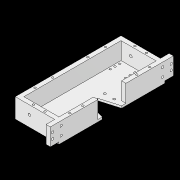
# Autodesk Inventor part: AfterComp1Chassis
Saved by Autodesk Inventor 2022 (Build 260153000, 153)
## iProperties
Created: 2021-02-15
Part Number: AfterComp1Chassis
Material: UHMW, White
Document SubType Name: Modeling
Designer: Esketitttttt
Density: 0.94 g/cm^3
Appearance: Smooth - White
Mass: 85.6235 g
Surface Area: 428.67 cm^2
Volume: 91.0888 cm^3
ThreadingScrew: 0.116 in
ThroughScrew: 0.138 in
Author: Esketitttttt
Autodesk Inventor part; units mm, degrees
ref_plane "YZ Plane" through (0, 0, 0) normal (1, 0, 0) x (0, 1, 0)
ref_plane "XZ Plane" through (0, 0, 0) normal (0, 1, 0) x (-1, 0, 0)
sketch "BasePlan" plane through (0, 0, 0) normal (0, 1, 0) x (-1, 0, 0)
  line L0 (0, 0) -> (-51.64, 0)
  line L1 (-51.64, 0) -> (-51.64, -28.5122)
  line L2 (-51.64, -28.5122) -> (0, -28.5122)
  line L3 (0, -28.5122) -> (0, 0)
  line L4 (0, 0) -> (-28.78, 0)
  line L5 (-28.78, 0) -> (-28.78, 57.15)
  line L6 (-28.78, 57.15) -> (0, 57.15)
  line L7 (0, 57.15) -> (0, 0)
  line L8 (-28.78, 57.15) -> (-51.64, 57.15)
  line L9 (-51.64, 57.15) -> (-51.64, 0)
  line L10 (-51.64, 0) -> (-28.78, 0)
  line L11 (-28.78, 0) -> (-28.78, 57.15)
  line L12 (0, 0) -> (0, -14.2561)
  line L13 (0, -14.2561) -> (8.9825, -14.2561) construction
  line L14 (-28.78, -28.5122) -> (-28.78, -85.6622)
  line L15 (-28.78, -85.6622) -> (0, -85.6622)
  line L16 (0, -85.6622) -> (0, -28.5122)
  line L17 (-28.78, -85.6622) -> (-51.64, -85.6622)
  line L18 (-51.64, -85.6622) -> (-51.64, -28.5122)
  line L19 (0, -85.6622) -> (6.35, -85.6622) construction
  line L20 (6.35, -85.6622) -> (6.35, -92.0122) construction
  line L21 (6.35, -92.0122) -> (0, -92.0122) construction
  line L22 (0, -92.0122) -> (0, -85.6622) construction
  line L23 (0, 57.15) -> (6.35, 57.15) construction
  line L24 (6.35, 57.15) -> (6.35, 63.5) construction
  line L25 (6.35, 63.5) -> (0, 63.5) construction
  line L26 (0, 63.5) -> (0, 57.15) construction
  line L27 (-51.64, -85.6622) -> (-57.99, -85.6622) construction
  line L28 (-57.99, -85.6622) -> (-57.99, -92.0122) construction
  line L29 (-57.99, -92.0122) -> (-51.64, -92.0122) construction
  line L30 (-51.64, -92.0122) -> (-51.64, -85.6622) construction
  line L31 (-51.64, 57.15) -> (-57.99, 57.15) construction
  line L32 (-57.99, 57.15) -> (-57.99, 63.5) construction
  line L33 (-57.99, 63.5) -> (-51.64, 63.5) construction
  line L34 (-51.64, 63.5) -> (-51.64, 57.15) construction
  line L35 (-57.99, 63.5) -> (-51.64, 63.5)
  line L36 (-51.64, 63.5) -> (-51.64, 0)
  line L37 (-51.64, 0) -> (-57.99, 0)
  line L38 (-57.99, 0) -> (-57.99, 63.5)
  line L39 (6.35, 63.5) -> (0, 63.5)
  line L40 (0, 63.5) -> (0, -92.0122)
  line L41 (0, -92.0122) -> (6.35, -92.0122)
  line L42 (6.35, -92.0122) -> (6.35, 63.5)
  line L43 (-51.64, 63.5) -> (0, 63.5)
  line L44 (0, 63.5) -> (0, 57.15)
  line L45 (0, 57.15) -> (-51.64, 57.15)
  line L46 (-51.64, 57.15) -> (-51.64, 63.5)
  line L47 (-51.64, -85.6622) -> (0, -85.6622)
  line L48 (0, -85.6622) -> (0, -92.0122)
  line L49 (0, -92.0122) -> (-51.64, -92.0122)
  line L50 (-51.64, -92.0122) -> (-51.64, -85.6622)
  line L51 (-57.99, -92.0122) -> (-51.64, -92.0122)
  line L52 (-51.64, -92.0122) -> (-51.64, -28.5122)
  line L53 (-51.64, -28.5122) -> (-57.99, -28.5122)
  line L54 (-57.99, -28.5122) -> (-57.99, -92.0122)
  line L55 (-51.64, -28.5122) -> (-57.99, -28.5122)
  line L56 (-57.99, -28.5122) -> (-57.99, -34.8622)
  line L57 (-57.99, -34.8622) -> (-51.64, -34.8622)
  line L58 (-51.64, -34.8622) -> (-51.64, -28.5122)
  line L59 (-51.64, 0) -> (-57.99, 0)
  line L60 (-57.99, 0) -> (-57.99, 6.35)
  line L61 (-57.99, 6.35) -> (-51.64, 6.35)
  line L62 (-51.64, 6.35) -> (-51.64, 0)
  line L63 (-51.64, 63.5) -> (-57.99, 63.5)
  line L64 (-57.99, 63.5) -> (-57.99, 76.2)
  line L65 (-57.99, 76.2) -> (-51.64, 76.2)
  line L66 (-51.64, 76.2) -> (-51.64, 63.5)
  line L67 (-57.99, -92.0122) -> (-51.64, -92.0122)
  line L68 (-57.99, -92.0122) -> (-57.99, -104.7122)
  line L69 (-57.99, -104.7122) -> (-51.64, -104.7122)
  line L70 (-51.64, -104.7122) -> (-51.64, -92.0122)
  line L71 (-51.64, -14.2561) -> (-31.066, -14.2561) construction
  line L72 (-31.066, -14.2561) -> (-31.066, -20.6061)
  line L73 (-31.066, -14.2561) -> (-31.066, -7.9061)
  line L74 (-57.99, 0) -> (-31.066, -7.9061)
  line L75 (-57.99, -28.5122) -> (-31.066, -20.6061)
  point P0 (0, -85.6622)
  point P1 (-51.64, 6.35)
  dimension "d3" = 28.78
  dimension "d5" = 22.86
  dimension "d6" = 28.5122
  dimension "d7" = 57.15
  dimension "d8" = 51.64
  dimension "d9" = 51.64
  dimension "d10" = 14.2561
  dimension "d12" = 6.35
  dimension "d88" = 6.35
  dimension "d89" = 6.35
  dimension "d90" = 6.35
  dimension "d158" = 155.5122
  dimension "d210" = 12.7
  dimension "d219" = 20.574
  dimension "d220" = 6.35
  dimension "d221" = 6.35
  constraints: 152 end point, 30 parallel, 17 horizontal, 15 perpendicular, 10 symmetric about line, 7 equal length, 4 point on line, 2 midpoint, 2 vertical
  measures "d3" distance of L5.end L6.end
  measures "d5" distance of L5.end L8.end
  measures "d6" distance of L2.end L0.start
  measures "d7" distance of L6.end L0.start
  measures "d8" distance of L8.end L6.end
  measures "d9" distance of L1.end L2.end
  measures "d10" distance of L0.start L12.end
  measures "d12" distance of L19.end L20.end
  measures "d88" distance of L57.end L56.end
  measures "d89" distance of L56.end L55.end
  measures "d90" distance of L59.end L60.end
  measures "d158" distance of L41.end L24.end
  measures "d210" distance of L63.end L64.end
  measures "d219" distance of L71.start L71.end
  measures "d220" distance of L71.end L72.end
  measures "d221" distance of L71.end L73.end
extrude "BackWall" add sketch "BasePlan" along normal blind 25.4 contours L7 L40 L39 L42 L41 L16 L3
sketch "Sketch2" plane through (-6.35, 0, -92.0122) normal (-1, 0, 0) x (0, 0, 1)
  line L0 (0, 0) -> (0, 25.4) construction
  line L1 (0, 0) -> (155.5122, 0) construction
  line L2 (0, 0) -> (3.175, 0) construction
  line L3 (3.175, 0) -> (3.175, 6.35) construction
  line L4 (3.175, 6.35) -> (0, 6.35) construction
  line L5 (0, 6.35) -> (0, 0) construction
  line L6 (3.175, 0) -> (3.175, 19.05) construction
  line L7 (0, 25.4) -> (155.5122, 25.4) projected
  line L8 (0, 25.4) -> (77.7561, 25.4) construction
  line L9 (77.7561, 25.4) -> (77.7561, 53.975) construction
  point P0 (92.0122, 0)
  point P1 (6.35, 0)
  point P2 (152.3372, 19.05)
  point P3 (152.3372, 6.35)
  dimension "d25" = 6.35
  dimension "d26" = 25.4
  dimension "d27" = 3.175
  dimension "d28" = 6.35
  dimension "d29" = 19.05
  dimension "d30" = 155.5122
  dimension "d31" = 77.7561
  constraints: 14 end point, 2 coincident, 2 parallel, 2 symmetric about line, 1 horizontal, 1 midpoint, 1 perpendicular, 1 point on line, 1 vertical
  measures "d25" distance of L0.start point (6.35, 0)
  measures "d26" distance of L0.start L0.end
  measures "d27" distance of L4.end L3.end
  measures "d28" distance of L3.end L2.end
  measures "d29" distance of L2.end L6.end
  measures "d30" distance of L0.end L7.end
  measures "d31" distance of L0.end L8.end
extrude "LeftSideWall" add sketch "BasePlan" along normal up to surface (25.4 mm away) contours L40 L49 L50 L17 L15
extrude "RightSideWall" add sketch "BasePlan" along normal up to surface (25.4 mm away) contours L6 L8 L36 L43 L40
hole "BackHoles" at (-6.35, 6.35, -88.8372) at (-6.35, 19.05, -88.8372) at (-6.35, 19.05, 60.325) at (-6.35, 6.35, 60.325) direction (1, 0, 0) diameter 3.5052 depth 6.35
hole "Back Threading Holes" at (-6.35, 6.35, -88.8372) at (-6.35, 19.05, -88.8372) at (-6.35, 19.05, 60.325) at (-6.35, 6.35, 60.325) direction (1, 0, 0) diameter 2.9464 depth 12.7 tip angle 118
extrude "RightFrontWall" add sketch "BasePlan" along normal up to surface (25.4 mm away) contours L61 L38 L35 L36 L9 | L35 L64 L65 L66
extrude "LeftFrontWall" add sketch "BasePlan" along normal up to surface (25.4 mm away) contours L18 L50 L51 L54 L57 | L70 L69 L68 L51
extrude "BottomUHMW" add sketch "BasePlan" against normal blind 3.175 contours L3 L2 L1 L75 L72 L73 L74 L0 | L7 L40 L39 L42 L41 L16 L3 | L0 L5 L6 L7 | L0 L9 L8 L5 | L6 L8 L36 L43 L40 | L37 L38 L61 L9 | L1 L74 L37 | L16 L15 L14 L2 | L61 L38 L35 L36 L9 | L14 L17 L18 L2 | L40 L49 L50 L17 L15 | L1 L53 L75 | L18 L57 L54 L53 | L18 L50 L51 L54 L57
sketch "Sketch4" plane through (0, 25.4, 0) normal (0, -1, 0) x (1, 0, 0)
  line L0 (-4.7625, -65.2173) -> (-4.7625, -63.6933) construction
  line L1 (-4.7625, -65.2173) -> (-4.7625, -63.6933) construction
  line L2 (0, -92.0122) -> (0, -85.6622) construction
  line L3 (-6.35, -81.3497) -> (-6.35, -92.0122) construction
  line L4 (-6.35, -76.5872) -> (-6.35, -81.3497) construction
  line L5 (0, 57.15) -> (0, -85.6622)
  line L6 (0, -14.2561) -> (-6.35, -14.2561)
  line L7 (54.815, -34.8622) -> (57.99, -34.8622) construction
  line L8 (57.99, -34.8622) -> (57.99, -53.9122) construction
  line L9 (57.99, -53.9122) -> (54.815, -53.9122) construction
  line L10 (54.815, -53.9122) -> (54.815, -34.8622) construction
  line L11 (54.815, -77.7247) -> (54.815, -72.9622) construction
  line L12 (-6.35, -92.0122) -> (57.99, -92.0122)
  line L13 (-6.35, -92.0122) -> (57.99, -92.0122) projected
  line L14 (-6.35, -92.0122) -> (-3.175, -92.0122)
  line L15 (-3.175, -92.0122) -> (-3.175, -66.0935) construction
  line L16 (51.64, -85.6622) -> (0, -85.6622) projected
  line L17 (-3.175, -92.0122) -> (-3.175, -40.1748) construction
  line L18 (57.99, -92.0122) -> (57.99, -28.5122) projected
  line L19 (57.99, -34.8622) -> (51.64, -34.8622) projected
  line L20 (57.99, 63.5) -> (51.64, 63.5) projected
  point P0 (0, 0)
  point P1 (-7.579, 35.8142)
  point P2 (-3.175, 37.5813)
  point P3 (51.64, -92.0122)
  point P4 (-3.175, 11.6626)
  point P5 (57.99, 25.4)
  point P6 (54.815, 44.45)
  point P7 (57.99, -30.9122)
  point P8 (51.3867, -22.9506)
  point P9 (54.815, 25.4)
  point P10 (-6.35, 63.5)
  dimension "d91" = 3.175
  dimension "d104" = 4.7625
  dimension "d118" = 3.175
  dimension "d119" = 25.9187
  dimension "d121" = 77.7561
  dimension "d132" = 51.8374
  dimension "d160" = 57.15
  dimension "d161" = 19.05
  dimension "d162" = 19.05
  dimension "d195" = 0
  dimension "d199" = 155.5122
  constraints: 32 end point, 6 coincident, 5 point on line, 5 symmetric about line, 2 parallel, 2 perpendicular, 1 horizontal, 1 midpoint, 1 vertical, 3 other
  measures "d91" distance of L8.end L9.end
  measures "d104" distance of L11.start L11.end
  measures "d118" distance of L3.end L14.end
  measures "d119" distance of L14.end L15.end
  measures "d121" distance between parallel lines of L12 L6
  measures "d132" distance of L14.end L17.end
  measures "d160" vertical distance of L7.end point (51.64, -92.012)
  measures "d161" vertical distance of point (54.815, -72.962) point (51.64, -92.012)
  measures "d162" distance of L7.end point (57.99, -53.912)
  measures "d195" distance between parallel lines of L10 L11
  measures "d199" distance between parallel lines of L20 L13
hole "NewTopHoles" at (-3.175, 25.4, 37.5813) at (-3.175, 25.4, -66.0935) at (54.815, 25.4, -72.9622) at (-3.175, 25.4, -40.1748) at (-3.175, 25.4, 11.6626) at (54.815, 25.4, 44.45) at (54.815, 25.4, -53.9122) at (54.815, 25.4, 25.4) direction (0, -1, 0) diameter 2.9464 depth 12.7 tip angle 118
sketch "Sketch5" plane through (0, 25.4, 0) normal (0, 1, 0) x (1, 0, 0)
  line L0 (-6.35, -63.5) -> (-1.5875, -63.5) construction
  line L1 (-1.5875, -63.5) -> (-1.5875, -58.7375) construction
  line L2 (-1.5875, -58.7375) -> (-6.35, -58.7375) construction
  line L3 (-6.35, -58.7375) -> (-6.35, -63.5) construction
  line L4 (-6.35, -58.7375) -> (-3.9687, -58.7375) construction
  line L5 (-3.9687, -58.7375) -> (-3.9687, -53.975) construction
  line L6 (-3.9687, -53.975) -> (-6.35, -53.975) construction
  line L7 (-6.35, -53.975) -> (-6.35, -58.7375) construction
  line L8 (23.9254, -63.0415) -> (25.7232, -67.4516)
  line L9 (20.7687, 14.2561) -> (-4.7625, 14.2561)
  line L10 (-6.35, -63.5) -> (51.64, -63.5) projected
  line L11 (-6.35, 92.0122) -> (-6.35, -63.5) projected
  line L12 (-6.35, 14.2561) -> (-15.875, 14.2561)
  line L13 (37.5312, -37.0575) -> (37.5312, -32.295) construction
  line L14 (-57.8724, 60.5133) -> (-57.8724, 55.7508) construction
  circle A0 centre (54.815, 71.1289) radius 1.4732 projected
  circle A1 centre (38.8013, -32.295) radius 1.0922 projected
  point P0 (0, 0)
  point P1 (-3.9688, 82.4872)
  point P2 (-3.9688, 82.4872)
  point P3 (57.99, -63.5)
  dimension "d63" = 17.7775
  dimension "d64" = 2.3813
  dimension "d65" = 4.7625
  dimension "d66" = 0
  dimension "d106" = 4.7625
  dimension "d107" = 4.7625
  constraints: 26 end point, 6 symmetric about line, 4 coincident, 4 parallel, 3 horizontal, 2 perpendicular, 2 vertical, 2 other
  measures "d64" distance of L6.end L5.end
  measures "d65" distance of L5.end L4.end
  measures "d66" distance between parallel lines of L12 L9
  measures "d106" distance of L13.start L13.end
  measures "d107" distance of L14.start L14.end
hole "TopHoles" [suppressed]
sketch "Sketch6" plane through (57.99, 1.5875, 96.9182) normal (1, 0, 0) x (0, 0, -1)
  line L0 (33.4182, -1.5875) -> (33.4182, 23.8125) construction
  line L1 (0, 0) -> (146.8373, -1.5875) construction
  line L2 (33.4182, -1.5875) -> (36.5932, -1.5875) construction
  line L3 (36.5932, -1.5875) -> (36.5932, 4.7625) construction
  line L4 (36.5932, 4.7625) -> (33.4182, 4.7625) construction
  line L5 (33.4182, 4.7625) -> (33.4182, -1.5875) construction
  line L6 (36.5932, -1.5875) -> (36.5932, 17.4625) construction
  line L7 (33.4182, 23.8125) -> (188.9304, 23.8125)
  line L8 (0, 25.4) -> (57.8525, 25.4) construction
  line L9 (57.8525, 25.4) -> (57.8525, 53.975) construction
  line L10 (111.1743, 23.8125) -> (111.1743, 30.162)
  line L11 (191.3304, -1.5875) -> (191.3304, -4.7625) projected
  line L12 (33.4182, -1.5875) -> (33.4182, -4.7625) projected
  point P0 (66.8365, 0)
  point P1 (27.0699, -1.4434)
  point P2 (146.8372, -1.5875)
  point P3 (0, 0)
  point P4 (185.7554, 17.4625)
  point P5 (185.7554, 4.7625)
  point P6 (188.9304, -4.7625)
  point P7 (188.9304, -1.5875)
  dimension "d85" = 6.35
  dimension "d86" = 25.4
  dimension "d77" = 3.175
  dimension "d78" = 6.35
  dimension "d76" = 19.05
  dimension "d75" = 57.8525
  dimension "d164" = 157.9122
  constraints: 20 end point, 3 vertical, 2 coincident, 2 parallel, 2 symmetric about line, 1 horizontal, 1 midpoint, 1 perpendicular, 1 point on line, 4 other
  measures "d85" distance of L0.start point (27.07, -1.443)
  measures "d86" distance of L0.end L0.start
  measures "d77" distance of L4.end L3.end
  measures "d78" distance of L3.end L2.end
  measures "d76" distance of L2.end L6.end
  measures "d75" distance of L8.start L8.end
hole "Front Holes" at (57.99, 6.35, 60.325) at (57.99, 19.05, 60.325) at (57.99, 19.05, -88.8372) at (57.99, 6.35, -88.8372) direction (-1, 0, 0) diameter 3.5052 depth 6.35
hole "Front Threading Holes" at (57.99, 19.05, 60.325) at (57.99, 6.35, 60.325) at (57.99, 6.35, -88.8372) at (57.99, 19.05, -88.8372) direction (-1, 0, 0) diameter 2.9464 depth 12.7 tip angle 118
sketch "Sketch7" plane through (51.64, 25.4, 57.15) normal (0, 0, -1) x (-1, 0, 0)
  line L0 (37.25, -22.225) -> (37.25, -12.7) construction
  line L1 (37.25, -12.7) -> (51.64, -12.7) construction
  line L2 (51.64, -12.7) -> (51.64, -25.4)
  circle A0 centre (37.25, -12.7) radius 8.04 construction
  circle A1 centre (37.25, -12.7) radius 2.96
  line L3 (37.25, -12.7) -> (37.25, -7.2) construction
  line L4 (37.25, -12.7) -> (37.25, -18.2) construction
  circle A2 centre (37.25, -18.2) radius 1.143
  circle A3 centre (37.25, -7.2) radius 1.143
  circle A4 centre (37.25, -12.7) radius 2
  line L5 (35.15, -9.525) -> (27.11, -9.525) construction
  line L6 (51.64, 0) -> (51.64, -25.4) projected
  dimension "d93" = 14.39
  dimension "d94" = 5.5
  dimension "d95" = 5.5
  dimension "d96" = 2.286
  dimension "d97" = 2.286
  dimension "d98" = 4
  dimension "d101" = 12.7
  dimension "d194" = 0
  constraints: 12 end point, 5 centre point, 5 coincident, 1 horizontal, 1 parallel, 1 vertical
  measures "d93" distance of L3.start L1.end
  measures "d94" distance of L3.start L3.end
  measures "d95" distance of L3.start L4.end
  measures "d96" diameter of A2
  measures "d97" diameter of A3
  measures "d98" diameter of A4
  measures "d101" distance of L1.end L2.end
  measures "d194" distance between parallel lines of L2 L6
extrude "MotorHole" cut sketch "Sketch7" along normal through all both and the other way through all contours A4
sketch "Sketch8" plane through (0, -3.175, 0) normal (0, -1, 0) x (1, 0, 0)
  line L0 (16.238, -28.5122) -> (16.238, -34.8622)
  line L1 (16.238, -31.6872) -> (30.1553, -31.6872) construction
  line L2 (30.1553, -31.6872) -> (44.0727, -31.6872) construction
  line L3 (57.99, -28.5122) -> (57.99, 0)
  line L4 (57.99, -14.2561) -> (39.7101, -14.2561)
  line L5 (16.238, 3.175) -> (30.1553, 3.175) construction
  line L6 (30.1553, 3.175) -> (44.0727, 3.175) construction
  line L7 (57.99, -34.8622) -> (51.64, -34.8622) projected
  line L8 (16.238, -34.8622) -> (57.99, -34.8622)
  line L9 (57.99, -92.0122) -> (57.99, -28.5122) projected
  point P0 (0, 0)
  point P1 (0, 44.9224)
  point P2 (51.64, -37.2622)
  point P3 (57.99, 0)
  dimension "d109" = 13.9173
  dimension "d110" = 13.9173
  dimension "d196" = 3.175
  dimension "d197" = 3.175
  dimension "d198" = 3.175
  dimension "d200" = 13.9173
  constraints: 16 end point, 5 coincident, 5 symmetric about line, 2 horizontal, 2 midpoint, 2 vertical, 1 other
  measures "d109" distance of L1.start L1.end
  measures "d110" distance of L1.end L2.end
  measures "d196" distance from line of L8 L2.end
  measures "d197" distance from line of point (30.155, -31.687) L8
  measures "d198" distance of L0.end L1.start
  measures "d200" distance from line of L9 L2.end
hole "UprightHoles" at (30.1553, -3.175, -31.6872) at (44.0727, -3.175, -31.6872) at (44.0727, -3.175, 3.175) at (30.1553, -3.175, 3.175) direction (0, 1, 0) diameter 3.5052 depth 9.525 tip angle 118
sketch "Sketch9" plane through (0, 25.4, 0) normal (0, -1, 0) x (1, 0, 0)
  line L0 (0, 57.15) -> (51.64, 57.15) construction
  line L1 (51.64, -85.6622) -> (0, -85.6622) construction
  line L2 (-6.35, -92.0122) -> (51.64, -92.0122) construction
  line L3 (-6.35, 63.5) -> (51.64, 63.5) construction
  line L4 (51.64, 57.15) -> (51.64, 6.35) construction
  line L5 (0, 57.15) -> (0, -85.6622) construction
  line L6 (0, -85.6622) -> (51.64, -85.6622) construction
  line L7 (-6.35, -92.0122) -> (57.99, -92.0122) construction
  line L8 (0, -85.6622) -> (0, -92.0122) construction
  line L9 (0, 57.15) -> (0, 63.5) construction
  line L10 (57.99, 63.5) -> (-6.35, 63.5) construction
  line L11 (51.64, 57.15) -> (51.64, 63.5) construction
  line L12 (51.64, -88.8372) -> (34.4267, -88.8372) construction
  line L13 (34.4267, -88.8372) -> (17.2133, -88.8372) construction
  line L14 (0, -14.2561) -> (7.9375, -14.2561)
  line L15 (-6.35, 63.5) -> (-6.35, -92.0122) projected
  point P0 (0, 0)
  point P1 (17.2133, 60.325)
  point P2 (34.4267, 60.325)
  dimension "d123" = 17.2133
  dimension "d124" = 17.2133
  dimension "d163" = 6.35
  dimension "d222" = 51.64
  dimension "d223" = 3.175
  dimension "d224" = 6.35
  constraints: 14 end point, 5 point on line, 2 coincident, 2 horizontal, 2 perpendicular, 2 symmetric about line, 1 midpoint, 1 parallel, 1 vertical alignment
  measures "d123" distance of L12.start L12.end
  measures "d124" distance of L12.end L13.end
  measures "d163" distance from line of L15 L1.end
  measures "d222" distance of L1.start L1.end
  measures "d223" distance from line of L7 point (17.213, -88.837)
  measures "d224" distance between parallel lines of L7 L1
hole "SideWallTopHoles" at (17.2133, 25.4, -88.8372) at (34.4267, 25.4, -88.8372) at (17.2133, 25.4, 60.325) at (34.4267, 25.4, 60.325) direction (0, -1, 0) diameter 2.9464 depth 9.525 tip angle 118
ref_plane "MidHeightPlane" through (0, 11.1125, 0) normal (0, 1, 0) x (1, 0, 0)
sketch "Sketch10" plane through (57.99, 25.4, 63.5) normal (1, 0, 0) x (0, 0, -1)
  circle A0 centre (9.525, -16.9333) radius 1.0922
  circle A1 centre (9.525, -8.4667) radius 1.0922
  circle A2 centre (53.975, -8.4667) radius 1.0922
  circle A3 centre (53.975, -16.9333) radius 1.0922
  circle A4 centre (101.5372, -16.9333) radius 1.0922
  circle A5 centre (101.5372, -8.4667) radius 1.0922
  circle A6 centre (148.3872, -8.4667) radius 1.0922
  circle A7 centre (148.3872, -16.9333) radius 1.0922
  line L0 (41.82, 0) -> (0, 0)
  line L1 (114.519, 0) -> (72.699, 0)
  line L2 (57.15, 0) -> (-12.7, 0) projected
  line L3 (0, -25.4) -> (0, -28.575) projected
  line L4 (57.15, -25.4) -> (57.15, 0) projected
  line L5 (98.3622, -25.4) -> (98.3622, 0) projected
  line L6 (157.9122, -25.4) -> (157.9122, -28.575) projected
  line L7 (168.2122, 0) -> (100.7622, 0) projected
  circle A8 centre (-9.525, -8.4667) radius 1.0922
  circle A9 centre (-9.525, -16.9333) radius 1.0922
  circle A10 centre (165.0372, -8.4667) radius 1.0922
  circle A11 centre (165.0372, -16.9333) radius 1.0922
  line L8 (-12.7, -25.4) -> (-12.7, 0) projected
  point P0 (100.7622, -25.4)
  point P1 (155.5122, -28.575)
  point P2 (157.9122, 0)
  point P3 (155.5122, -25.4)
  point P4 (98.3622, 0)
  dimension "d167" = 9.525
  dimension "d168" = 9.525
  dimension "d169" = 3.175
  dimension "d170" = 3.175
  dimension "d171" = 8.4667
  dimension "d172" = 8.4667
  dimension "d173" = 3.175
  dimension "d174" = 3.175
  dimension "d175" = 9.525
  dimension "d176" = 9.525
  dimension "d177" = 8.4667
  dimension "d178" = 8.4667
  dimension "d179" = 8.4667
  dimension "d180" = 2.1844
  dimension "d181" = 2.1844
  dimension "d182" = 2.1844
  dimension "d183" = 2.1844
  dimension "d184" = 2.1844
  dimension "d185" = 2.1844
  dimension "d186" = 2.1844
  dimension "d187" = 2.1844
  dimension "d208" = 25.4
  dimension "d209" = 28.575
  dimension "d211" = 2.1844
  dimension "d212" = 2.1844
  dimension "d213" = 2.1844
  dimension "d214" = 2.1844
  dimension "d215" = 8.4667
  dimension "d216" = 8.4667
  dimension "d217" = 3.175
  dimension "d218" = 3.175
  constraints: 12 centre point, 5 horizontal alignment, 4 coincident, 4 end point, 2 vertical alignment, 2 other
  measures "d167" distance from line of L3 A1.centre
  measures "d168" distance from line of L3 A0.centre
  measures "d169" distance from line of A2.centre L4
  measures "d170" distance from line of L4 A3.centre
  measures "d171" distance of A3.centre A2.centre
  measures "d172" distance of A0.centre A1.centre
  measures "d177" distance of A7.centre A6.centre
  measures "d178" distance from line of L2 A1.centre
  measures "d179" distance from line of L7 A6.centre
  measures "d180" diameter of A7
  measures "d181" diameter of A6
  measures "d182" diameter of A5
  measures "d183" diameter of A4
  measures "d184" diameter of A3
  measures "d185" diameter of A2
  measures "d186" diameter of A0
  measures "d187" diameter of A1
  measures "d208" distance of L4.start L2.start
  measures "d209" distance of point (0, 0) L3.end
  measures "d211" diameter of A8
  measures "d212" diameter of A9
  measures "d213" diameter of A10
  measures "d214" diameter of A11
  measures "d215" distance from line of L2 A8.centre
  measures "d216" distance of A9.centre A8.centre
  measures "d217" distance from line of L8 A8.centre
  measures "d218" horizontal distance of L7.start A10.centre
hole "WedgeletHoles" at (57.99, 16.9333, -101.5372) at (57.99, 8.4667, -101.5372) at (57.99, 8.4667, 73.025) at (57.99, 16.9333, 73.025) direction (-1, 0, 0) diameter 3.5052 depth 6.35 tip angle 118
sketch "Sketch11" plane through (0, -3.175, 0) normal (0, -1, 0) x (1, 0, 0)
  line L0 (-6.35, -92.0122) -> (-6.35, 63.5) projected
  line L1 (-6.35, 63.5) -> (57.99, 63.5)
  line L2 (57.99, 63.5) -> (57.99, -92.0122)
  line L3 (51.64, -85.6622) -> (51.64, 57.15)
  line L4 (51.64, 57.15) -> (0, 57.15)
  line L5 (0, 57.15) -> (0, -85.6622)
  line L6 (0, -85.6622) -> (51.64, -85.6622)
  line L7 (28.78, 33.15) -> (0, 33.15) construction
  line L8 (0, 33.15) -> (0, 57.15)
  line L9 (28.78, 33.15) -> (28.78, 45.15)
  line L10 (0, 45.15) -> (0, 33.15)
  line L11 (28.78, 33.15) -> (28.78, 57.15)
  line L12 (28.78, 32.995) -> (28.78, 57.15)
  line L13 (28.78, 33.15) -> (28.78, 39.15)
  line L14 (28.78, 57.15) -> (0, 57.15)
  line L15 (51.64, 2.4) -> (51.64, -30.9122)
  line L16 (51.64, -14.2561) -> (32.0322, -14.2561)
  line L17 (51.64, -14.2561) -> (71.2478, -14.2561) construction
  line L18 (0, 33.15) -> (3.175, 33.15)
  line L19 (28.78, 33.15) -> (25.605, 33.15)
  line L20 (25.605, 33.15) -> (25.605, 45.15) construction
  line L21 (14.39, 33.15) -> (14.39, 36.15) construction
  line L22 (25.605, 45.15) -> (25.605, 38.275) construction
  line L23 (25.605, 45.15) -> (25.605, 52.025) construction
  line L24 (-6.35, -92.0122) -> (57.99, -92.0122) projected
  line L25 (-6.35, -92.0122) -> (57.99, -92.0122)
  point P0 (0, 0)
  point P1 (3.175, 52.025)
  point P2 (3.175, 45.15)
  point P3 (3.175, 38.275)
  point P4 (25.605, -80.5372)
  point P5 (25.605, -80.5372)
  point P6 (25.605, -73.6622)
  point P7 (25.605, -66.7872)
  point P8 (3.175, -66.7872)
  point P9 (3.175, -73.6622)
  point P10 (3.175, -80.5372)
  dimension "d140" = 6.35
  dimension "d150" = 180
  dimension "d189" = 0
  dimension "d190" = 0
  dimension "d201" = 28.78
  dimension "d202" = 24
  dimension "d203" = 3.175
  dimension "d204" = 3.175
  dimension "d205" = 12
  dimension "d206" = 6.875
  dimension "d207" = 6.875
  dimension "d225" = 6.35
  constraints: 48 end point, 10 symmetric about line, 5 coincident, 5 midpoint, 4 equal length, 4 vertical, 3 perpendicular, 3 point on line, 2 horizontal, 1 collinear, 1 other
  measures "d140" distance between parallel lines of L2 L3
  measures "d150" angle of L16 L17
  measures "d189" distance between parallel lines of L4 L14
  measures "d190" distance between parallel lines of L5 L8
  measures "d201" distance between parallel lines of L13 L5
  measures "d202" distance between parallel lines of L14 L7
  measures "d203" distance of L10.end L18.end
  measures "d204" distance of L11.start L19.end
  measures "d205" distance of L19.end L20.end
  measures "d206" distance of L20.end L22.end
  measures "d207" distance of L20.end L23.end
  measures "d225" distance between parallel lines of L6 L24
hole "BottomMotorMountHoles" at (25.605, -3.175, 52.025) at (25.605, -3.175, 45.15) at (25.605, -3.175, 38.275) at (3.175, -3.175, 52.025) at (3.175, -3.175, 45.15) at (3.175, -3.175, 38.275) at (3.175, -3.175, -66.7872) at (3.175, -3.175, -73.6622) at (3.175, -3.175, -80.5372) at (25.605, -3.175, -80.5372) at (25.605, -3.175, -73.6622) at (25.605, -3.175, -66.7872) direction (0, 1, 0) diameter 3 depth 9.525 tip angle 118
sketch "Sketch16" plane through (0, -3.175, 0) normal (0, -1, 0) x (1, 0, 0)
  circle A0 centre (17.2133, 60.325) radius 1.4732 construction
  circle A1 centre (17.2133, -88.8372) radius 1.4732 construction
  circle A2 centre (34.4267, -88.8372) radius 1.4732 construction
  circle A3 centre (34.4267, 60.325) radius 1.4732 construction
  circle A4 centre (54.815, -53.9122) radius 1.4732 construction
  circle A5 centre (-3.175, 11.6626) radius 1.4732 construction
  circle A6 centre (54.815, -72.9622) radius 1.4732 construction
  circle A7 centre (-3.175, 37.5813) radius 1.4732 construction
  circle A8 centre (-3.175, -66.0935) radius 1.4732 construction
  circle A9 centre (-3.175, -40.1748) radius 1.4732 construction
  circle A10 centre (54.815, 44.45) radius 1.4732 construction
  circle A11 centre (54.815, 25.4) radius 1.4732 construction
  line L0 (-6.35, -92.0122) -> (-6.35, 63.5) construction
  line L1 (-6.35, 63.5) -> (51.64, 63.5) construction
  line L2 (51.64, 76.2) -> (51.64, 63.5) construction
  line L3 (57.99, 76.2) -> (51.64, 76.2) construction
  line L4 (57.99, 6.35) -> (57.99, 76.2) construction
  line L5 (51.64, 6.35) -> (57.99, 6.35) construction
  line L6 (51.64, 57.15) -> (51.64, 6.35) construction
  line L7 (0, 57.15) -> (51.64, 57.15) construction
  line L8 (0, 57.15) -> (0, -85.6622) construction
  line L9 (51.64, -85.6622) -> (0, -85.6622) construction
  line L10 (51.64, -34.8622) -> (51.64, -85.6622) construction
  line L11 (57.99, -34.8622) -> (51.64, -34.8622) construction
  line L12 (57.99, -104.7122) -> (57.99, -34.8622) construction
  line L13 (51.64, -104.7122) -> (57.99, -104.7122) construction
  line L14 (51.64, -92.0122) -> (51.64, -104.7122) construction
  line L15 (-6.35, -92.0122) -> (51.64, -92.0122) construction
  line L16 (0, -90.5898) -> (0, -87.0846) construction
  line L17 (51.64, -87.0846) -> (51.64, -90.5898) construction
  line L18 (44.2369, -88.8372) -> (54.815, -88.8372) construction
  line L19 (7.4031, -88.8372) -> (-3.175, -88.8372) construction
  circle A12 centre (34.4267, -88.8372) radius 1.4732 construction
  circle A13 centre (54.815, -72.9622) radius 1.4732 construction
  line L20 (54.815, -72.9622) -> (54.815, -88.8372) construction
  line L21 (-3.175, -88.8372) -> (-3.175, -66.0935) construction
  line L22 (0, 57.15) -> (0, -85.6622) projected
  line L23 (0, -14.2561) -> (6.35, -14.2561)
  circle A14 centre (-3.175, -66.0935) radius 1.4732 construction
  circle A15 centre (-3.175, -40.1748) radius 1.4732 construction
  line L24 (-3.175, -66.0935) -> (-3.175, -40.1748) construction
  circle A16 centre (-3.175, 11.6626) radius 1.4732 construction
  line L25 (-3.175, -40.1748) -> (-3.175, 11.6626) construction
  line L26 (54.815, -72.9622) -> (54.815, -53.9122) construction
  line L27 (54.815, -53.9122) -> (54.815, -34.8622) construction
  line L28 (51.64, -34.8622) -> (57.99, -34.8622) construction
  circle A17 centre (17.2133, -88.8372) radius 1.4732 projected
  line L29 (15.7401, -88.8372) -> (7.4031, -88.8372)
  line L30 (0, -90.5898) -> (0, -87.0846) projected
  line L31 (44.2369, -88.8372) -> (35.8999, -88.8372) construction
  circle A18 centre (34.4267, -88.8372) radius 1.4732 projected
  point P0 (0, 0)
  point P1 (-3.175, -77.4653)
  point P2 (54.815, -80.8997)
  point P3 (40.0684, -88.8372)
  point P4 (11.5716, -88.8372)
  point P5 (-3.175, 48.9532)
  point P6 (54.815, 52.3875)
  point P7 (40.0684, 60.325)
  point P8 (11.5716, 60.325)
  point P9 (54.815, -63.4372)
  point P10 (54.815, -44.3872)
  point P11 (-3.175, -53.1341)
  point P12 (-3.175, -14.2561)
  point P13 (54.815, 34.925)
  point P14 (54.815, 15.875)
  point P15 (-3.175, 24.622)
  constraints: 22 end point, 10 midpoint, 7 symmetric about line, 4 horizontal, 3 vertical, 2 horizontal alignment, 2 perpendicular, 2 vertical alignment, 1 collinear, 2 other
hole "BottomHoles" at (-3.175, -3.175, -77.4653) at (54.815, -3.175, -80.8997) at (40.0684, -3.175, -88.8372) at (11.5716, -3.175, -88.8372) at (-3.175, -3.175, 48.9532) at (11.5716, -3.175, 60.325) at (40.0684, -3.175, 60.325) at (54.815, -3.175, 52.3875) at (54.815, -3.175, -63.4372) at (54.815, -3.175, -44.3872) at (-3.175, -3.175, -53.1341) at (-3.175, -3.175, -14.2561) at (-3.175, -3.175, 24.622) at (54.815, -3.175, 15.875) at (54.815, -3.175, 34.925) direction (0, 1, 0) diameter 3.5052 depth 3.175
hole "BottomThreadingHoles" at (54.815, -3.175, 52.3875) at (54.815, -3.175, 34.925) at (54.815, -3.175, 15.875) at (54.815, -3.175, -44.3872) at (54.815, -3.175, -63.4372) at (54.815, -3.175, -80.8997) at (40.0684, -3.175, 60.325) at (11.5716, -3.175, 60.325) at (-3.175, -3.175, -14.2561) at (-3.175, -3.175, 24.622) at (-3.175, -3.175, 48.9532) at (-3.175, -3.175, -53.1341) at (-3.175, -3.175, -77.4653) at (11.5716, -3.175, -88.8372) at (40.0684, -3.175, -88.8372) direction (0, 1, 0) diameter 2.9464 depth 12.7 tip angle 118
equation "\"d9\" = d8"
equation "\"d10\" = 0.5 * d6"
equation "\"d27\" = 0.5 * d25"
equation "\"d28\" = 0.25 * d26"
equation "\"d29\" = 3 * d28"
equation "\"d31\" = 0.5 * d30"
equation "\"d77\" = 0.5 * d85"
equation "\"d78\" = 0.25 * d86"
equation "\"d76\" = 3 * d78"
equation "\"ThreadingScrew\" = 2.9464"
equation "\"ThroughScrew\" = 3.5052"
body "Solid1"
